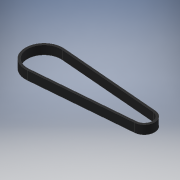
# Autodesk Inventor part: Cinghia
Saved by Autodesk Inventor 2018 (Build 220112000, 112)
## iProperties
Created: 2020-06-04
Part Number: Cinghia
Material: Gomma
Document SubType Name: Modeling
Designer: Francesco
Density: 0.93 g/cm^3
Appearance: Gomma - Nero
Author: Francesco
Autodesk Inventor part; units mm, degrees
ref_plane "YZ Plane" through (0, 0, 0) normal (1, 0, 0) x (0, 1, 0)
ref_plane "XZ Plane" through (0, 0, 0) normal (0, 1, 0) x (-1, 0, 0)
ref_plane "XY Plane" through (0, 0, 0) normal (0, 0, 1) x (1, 0, 0)
sketch "Schizzo1" plane through (0, 0, 0) normal (0, 0, 1) x (1, 0, 0)
  arc A0 (4.1667, 49.8261) -> (4.1667, -49.8261) centre (0, 0) ccw
  arc A1 (302.0833, -24.913) -> (302.0833, 24.913) centre (300, 0) ccw
  line L0 (4.1667, 49.8261) -> (302.0833, 24.913)
  line L1 (302.0833, -24.913) -> (4.1667, -49.8261)
  line L2 (302.5833, 30.8922) -> (4.6667, 55.8052)
  arc A2 (4.6667, 55.8052) -> (4.6667, -55.8052) centre (0, 0) ccw
  line L3 (4.6667, -55.8052) -> (302.5833, -30.8922)
  arc A3 (302.5833, -30.8922) -> (302.5833, 30.8922) centre (300, 0) ccw
  dimension "d0" = 100
  dimension "d1" = 50
  dimension "d2" = 300
  dimension "d3" = 6
  constraints: 8 end point, 8 point on circle, 4 centre point, 4 tangent, 1 coincident, 1 horizontal alignment, 3 other
  measures "d0" diameter of A0
  measures "d1" diameter of A1
  measures "d2" distance of point (0, 0) A1.centre
  measures "d3" distance between parallel lines of L0 L2
extrude "Estrusione1" add sketch "Schizzo1" along normal blind 26
